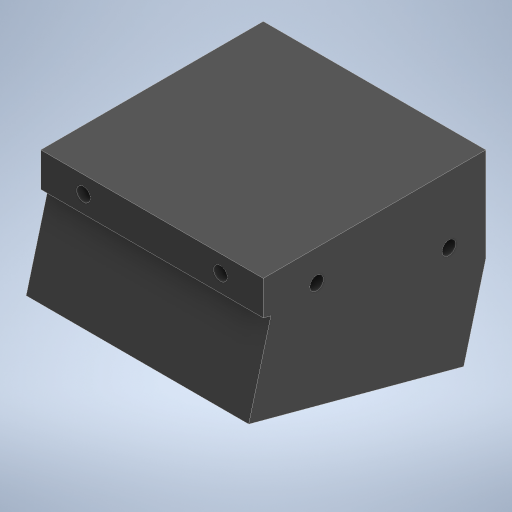
# Autodesk Inventor part: arm_middle
Saved by Autodesk Inventor 2024.1 (Build 281209000, 209)
## iProperties
Created: 2024-02-14
Part Number: arm_middle
Material: 一般
Document SubType Name: Modeling
Designer: hibik
Density: 1 g/cm^3
Appearance: 既定
Author: hibik
Autodesk Inventor part; units mm, degrees
ref_plane "YZ Plane" through (0, 0, 0) normal (1, 0, 0) x (0, 1, 0)
ref_plane "XZ Plane" through (0, 0, 0) normal (0, 1, 0) x (-1, 0, 0)
ref_plane "XY Plane" through (0, 0, 0) normal (0, 0, 1) x (1, 0, 0)
sketch "スケッチ3" plane through (0, 0, 0) normal (1, 0, 0) x (0, 1, 0)
  line L0 (0, 0) -> (10.9667, 0)
  line L1 (10.9667, 0) -> (10.9667, -26)
  line L2 (10.9667, -26) -> (0, -26)
  line L3 (0, -26) -> (0, 0)
  line L4 (10.9667, 0) -> (6.9667, 0)
  line L5 (6.9667, 0) -> (6.9667, -26)
  line L6 (6.9667, -26) -> (10.9667, -26)
  line L7 (10.9667, -26) -> (10.9667, 0)
  line L8 (6.9667, 0) -> (0, -26)
  point P0 (6.9667, 0)
  dimension "d3" = 26
  dimension "d4" = 4
  dimension "d5" = 15
  constraints: 18 end point, 4 parallel, 2 horizontal, 2 perpendicular, 1 point on line
  measures "d3" distance of L0.end L1.end
  measures "d4" distance between parallel lines of L1 L5
  measures "d5" angle of L5 L8
extrude "押し出し2" add sketch "スケッチ3" along normal blind 26 contours L0 L1 L2 L5 | L5 L2 L8
sketch "スケッチ4" plane through (0, 6.9667, 0) normal (0, 0, 1) x (1, 0, 0)
  line L0 (0, 4) -> (0, 0) projected
  line L1 (0, 0) -> (26, 0) projected
  line L2 (26, 4) -> (26, 0) projected
  line L3 (0, 4) -> (26, 4) projected
  circle A0 centre (5, 2) radius 0.8
  circle A1 centre (21, 2) radius 0.8
  point P0 (0, -6.9667)
  point P1 (0, 2)
  dimension "d8" = 1.6
  dimension "d9" = 1.6
  dimension "d10" = 5
  dimension "d11" = 5
  constraints: 2 centre point, 2 horizontal alignment, 1 midpoint
  measures "d8" diameter of A0
  measures "d9" diameter of A1
  measures "d10" distance from line of A0.centre L0
  measures "d11" distance from line of A1.centre L2
sketch "スケッチ5" plane through (26, 0, 0) normal (1, 0, 0) x (0, 0, -1)
  line L0 (0, 6.9667) -> (26, 0) projected
  line L1 (26, 0) -> (0.8859, 6.7293)
  line L2 (0.8859, 6.7293) -> (1.9212, 10.593)
  line L3 (1.9212, 10.593) -> (27.0353, 3.8637)
  line L4 (27.0353, 3.8637) -> (26, 0)
  circle A0 centre (21.688, 3.2259) radius 0.8
  circle A1 centre (6.2332, 7.3671) radius 0.8
  point P0 (0, 0)
  dimension "d14" = 4
  dimension "d15" = 26
  dimension "d16" = 1.6
  dimension "d17" = 1.6
  dimension "d18" = 2
  dimension "d19" = 2
  dimension "d20" = 5
  dimension "d21" = 5
  constraints: 8 end point, 2 centre point, 2 parallel, 1 perpendicular, 1 point on line
  measures "d14" distance between parallel lines of L0 L3
  measures "d15" distance between parallel lines of L4 L2
  measures "d16" diameter of A0
  measures "d17" diameter of A1
  measures "d18" distance from line of L3 A0.centre
  measures "d19" distance from line of L3 A1.centre
  measures "d20" distance from line of L2 A1.centre
  measures "d21" distance from line of L4 A0.centre
extrude "押し出し4" cut sketch "スケッチ5" against normal through all contours A0 | A1
extrude "押し出し8" cut sketch "スケッチ4" against normal through all contours A0 | A1
sketch "スケッチ8" plane through (26, 0, 0) normal (1, 0, 0) x (0, 0, -1)
  line L0 (26, 0) -> (26, 10.9667) projected
  line L1 (0, 6.9667) -> (26, 0) projected
  line L2 (26, 0) -> (0.8859, 6.7293)
  line L3 (0.8859, 6.7293) -> (-1.7023, -2.93)
  line L4 (-1.7023, -2.93) -> (23.4118, -9.6593)
  line L5 (23.4118, -9.6593) -> (26, 0)
  point P0 (0, 0)
  dimension "d39" = 26
  dimension "d40" = 10
  constraints: 8 end point, 2 parallel, 1 perpendicular, 1 point on line
  measures "d39" distance between parallel lines of L5 L3
  measures "d40" distance between parallel lines of L1 L4
extrude "押し出し9" add sketch "スケッチ8" against normal up to surface (26 mm away)
